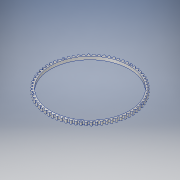
# Autodesk Inventor part: Turret Gear Large
Saved by Autodesk Inventor 2019.4 (Build 234330000, 330)
## iProperties
Created: 2020-01-12
Part Number: Turret Gear Large
Material: Aluminum 6061
Document SubType Name: Modeling
Designer: admin
Density: 2.7 g/cm^3
Appearance: Aluminum - Flat
Author: admin
Autodesk Inventor part; units mm, degrees
ref_plane "YZ Plane" through (0, 0, 0) normal (1, 0, 0) x (0, 1, 0)
ref_plane "XZ Plane" through (0, 0, 0) normal (0, 1, 0) x (-1, 0, 0)
ref_plane "XY Plane" through (0, 0, 0) normal (0, 0, 1) x (1, 0, 0)
sketch "Sketch1" plane through (0, 0, 0) normal (0, 1, 0) x (-1, 0, 0)
  circle A0 centre (0, 0) radius 127.5
  circle A1 centre (0, 0) radius 133.7014 construction
  line L0 (0, 0) -> (133.7014, 0) construction
  line L1 (133.5667, 5.9985) -> (0, 0) construction
  line L2 (133.5667, -5.9985) -> (0, 0) construction
  arc A2 (133.6341, 2.9992) -> (134.2989, 8.9078) centre (133.5667, 5.9985) ccw
  arc A3 (133.6341, 2.9992) -> (133.6341, -2.9992) centre (133.7014, 0) ccw
  arc A4 (133.3649, -8.9917) -> (133.6341, -2.9992) centre (133.5667, -5.9985) ccw
  arc A5 (133.3649, -8.9917) -> (132.8272, -14.966) centre (133.1631, -11.9849) ccw
  arc A6 (132.022, -20.9102) -> (132.8272, -14.966) centre (132.4913, -17.9472) ccw
  arc A7 (132.022, -20.9102) -> (130.951, -26.8123) centre (131.5527, -23.8733) ccw
  arc A8 (129.6162, -32.6604) -> (130.951, -26.8123) centre (130.3492, -29.7514) ccw
  arc A9 (129.6162, -32.6604) -> (128.0204, -38.4427) centre (128.8832, -35.5695) ccw
  arc A10 (126.1667, -44.1476) -> (128.0204, -38.4427) centre (127.1576, -41.316) ccw
  arc A11 (126.1667, -44.1476) -> (124.059, -49.7636) centre (125.1759, -46.9793) ccw
  arc A12 (121.7015, -55.2794) -> (124.059, -49.7636) centre (122.9421, -52.548) ccw
  arc A13 (121.7015, -55.2794) -> (119.0988, -60.6839) centre (120.4608, -58.0109) ccw
  arc A14 (116.2563, -65.9661) -> (119.0988, -60.6839) centre (117.7368, -63.3569) ccw
  arc A15 (116.2563, -65.9661) -> (113.1797, -71.1155) centre (114.7758, -68.5753) ccw
  arc A16 (109.8751, -76.1217) -> (113.1797, -71.1155) centre (111.5836, -73.6557) ccw
  arc A17 (109.8751, -76.1217) -> (106.3493, -80.9746) centre (108.1667, -78.5877) ccw
  arc A18 (102.6093, -85.6644) -> (106.3493, -80.9746) centre (104.5319, -83.3614) ccw
  arc A19 (102.6093, -85.6644) -> (98.6627, -90.1817) centre (100.6867, -87.9673) ccw
  arc A20 (94.5173, -94.5173) -> (98.6627, -90.1817) centre (96.6387, -92.396) ccw
  arc A21 (94.5173, -94.5173) -> (89.5795, -97.6717) centre (92.396, -96.6387) ccw
  line L3 (130.7014, 0) -> (127.5, 0)
  line L4 (130.1752, -11.716) -> (126.9867, -11.429)
  dimension "d3" = 267.4028
  dimension "d0" = 255
  dimension "d7" = 5.143
  dimension "d12" = 3
  dimension "d13" = 3
  dimension "d14" = 3
  dimension "d15" = 3
  dimension "d16" = 3
  dimension "d17" = 3
  dimension "d18" = 3
  dimension "d19" = 3
  dimension "d20" = 3
  dimension "d21" = 3
  dimension "d22" = 3
  dimension "d23" = 3
  dimension "d24" = 3
  dimension "d25" = 3
  dimension "d26" = 3
  dimension "d27" = 3
  dimension "d28" = 3
  dimension "d29" = 3
  dimension "d30" = 3
  dimension "d31" = 3
  constraints: 44 point on circle, 21 centre point, 19 equal radius, 10 end point, 2 coincident, 2 line through centre, 2 point on line, 1 horizontal, 23 other
  measures "d0" diameter of A0
  measures "d7" angle of L2 L1
  measures "d12" radius of A2
  measures "d13" radius of A3
  measures "d14" radius of A4
  measures "d15" radius of A5
  measures "d16" radius of A6
  measures "d17" radius of A7
  measures "d18" radius of A9
  measures "d19" radius of A8
  measures "d20" radius of A10
  measures "d21" radius of A11
  measures "d22" radius of A12
  measures "d23" radius of A13
  measures "d24" radius of A14
  measures "d25" radius of A15
  measures "d26" radius of A16
  measures "d27" radius of A17
  measures "d28" radius of A18
  measures "d29" radius of A19
  measures "d30" radius of A20
  measures "d31" radius of A21
extrude "Extrusion1" add sketch "Sketch1" along normal blind 10 contours L3 A3 A4 A5 L4 A0
pattern_circular "Circular Pattern1" count 70 over 360 about axis through (0, 0, 0) along (0, 1, 0) of "Extrusion1"
sketch "Sketch2" plane through (0, 10, 0) normal (0, 1, 0) x (1, 0, 0)
  circle A0 centre (0, 131.2014) radius 1.65
  arc A1 (2.9992, 133.6341) -> (-2.9992, 133.6341) centre (0, 133.7014) ccw construction
  line L0 (0, 131.2014) -> (0, 133.7014) construction
  point P0 (0, 0)
  dimension "d37" = 3.3
  dimension "d38" = 2.5
  constraints: 2 end point, 1 centre point, 1 vertical
  measures "d37" diameter of A0
  measures "d38" distance of L0.end L0.start
extrude "Extrusion2" cut sketch "Sketch2" against normal through all
pattern_circular "Circular Pattern2" count 5 over 360 about axis through (0, 0, 0) along (0, 1, 0) of "Extrusion2"
body "Solid1"
